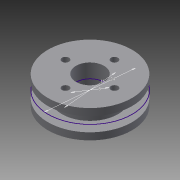
# Autodesk Inventor part: Servo Pulley
Saved by Autodesk Inventor 2015 (Build 190159000, 159)
## iProperties
Created: 2016-11-02
Part Number: Servo Pulley
Material: Generic
Document SubType Name: Modeling
Designer: Neelotpal Nag
Density: 1 g/cm^3
Appearance: Default
Author: Neelotpal Nag
Autodesk Inventor part; units mm, degrees
ref_plane "YZ Plane" through (0, 0, 0) normal (1, 0, 0) x (0, 1, 0)
ref_plane "XZ Plane" through (0, 0, 0) normal (0, 1, 0) x (-1, 0, 0)
ref_plane "XY Plane" through (0, 0, 0) normal (0, 0, 1) x (1, 0, 0)
sketch "Sketch1" plane through (0, 0, 0) normal (0, 0, 1) x (1, 0, 0)
  circle A0 centre (0, 0) radius 4
  circle A1 centre (0, 0) radius 8
  circle A2 centre (0, 0) radius 12
  dimension "d0" = 8
  dimension "d1" = 16
  dimension "d2" = 24
  constraints: 3 centre point, 3 coincident
  measures "d0" diameter of A0
  measures "d1" diameter of A1
  measures "d2" diameter of A2
extrude "Extrusion1" add sketch "Sketch1" along normal mid plane 4 contours A1
sketch "Sketch2" plane through (0, 0, 2) normal (0, 0, 1) x (1, 0, 0)
  circle A0 centre (0, 0) radius 12 projected
  circle A1 centre (0, 0) radius 8 projected
extrude "Extrusion2" add sketch "Sketch2" along normal blind 2 contours A0 | A1
mirror "Mirror1" about plane through (0, 0, 0) normal (0, 0, 1) of "Extrusion2"
extrude "Extrusion3" cut sketch "Sketch1" along normal through all both and the other way through all contours A0
sketch "Sketch3" plane through (0, 0, -4) normal (0, 0, -1) x (-1, 0, 0)
  circle A0 centre (0, 0) radius 7
  line L0 (0, -7) -> (0, 7)
  circle A1 centre (0, -7) radius 1
  circle A2 centre (0, 7) radius 1
  dimension "d9" = 14
  dimension "d10" = 2
  dimension "d11" = 2
  constraints: 3 centre point, 3 coincident, 2 end point, 2 point on circle, 1 vertical
  measures "d9" diameter of A0
  measures "d10" diameter of A1
  measures "d11" diameter of A2
extrude "Extrusion4" cut sketch "Sketch3" against normal through all contours A2 L0 A0 | A0 A2 | A1 A0 | A0 L0 A1 | L0 A2 A0 | A0 A1 L0
pattern_circular "Circular Pattern1" count 4 over 360 about axis through (0, 0, -10) along (0, 0, 1) of "Extrusion4"
body "Solid1"
